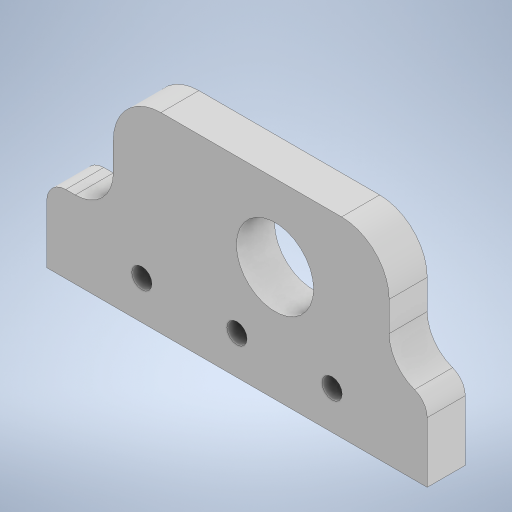
# Autodesk Inventor part: bottomhingeholder
Saved by Autodesk Inventor 2024 (Build 280153000, 153)
## iProperties
Created: 2023-09-15
Part Number: bottomhingeholder
Material: Generic
Document SubType Name: Modeling
Designer: komor
Density: 1 g/cm^3
Appearance: Default
Author: komor
Autodesk Inventor part; units mm, degrees
ref_plane "YZ Plane" through (0, 0, 0) normal (1, 0, 0) x (0, 1, 0)
ref_plane "XZ Plane" through (0, 0, 0) normal (0, 1, 0) x (-1, 0, 0)
ref_plane "XY Plane" through (0, 0, 0) normal (0, 0, 1) x (1, 0, 0)
sketch "Sketch1" plane through (0, 0, 0) normal (0, 0, 1) x (1, 0, 0)
  line L0 (30.5843, 30.8924) -> (30.5843, 10.8924)
  line L1 (30.5843, 10.8924) -> (-69.4157, 10.8924)
  line L2 (-69.4157, 10.8924) -> (-69.4157, 31.1924)
  line L3 (-69.4157, 21.0424) -> (30.5843, 20.8924) construction
  line L4 (-9.4157, 61.1924) -> (-39.4157, 61.1924)
  line L5 (-51.9157, 48.6924) -> (-51.9157, 41.1924)
  arc A0 (-39.4157, 61.1924) -> (-51.9157, 48.6924) centre (-39.4157, 48.6924) ccw
  line L6 (30.5843, 30.8924) -> (30.5843, 30.8924)
  line L7 (-61.9157, 31.1924) -> (-69.4157, 31.1924)
  arc A1 (-61.9157, 31.1924) -> (-51.9157, 41.1924) centre (-61.9157, 41.1924) ccw
  circle A2 centre (-19.4157, 20.9674) radius 2.65
  line L8 (-69.4157, 21.0424) -> (-19.4157, 20.9674) construction
  line L9 (-19.4157, 20.9674) -> (30.5843, 20.8924) construction
  circle A3 centre (-44.4157, 21.0049) radius 2.65
  circle A4 centre (5.5843, 20.9299) radius 2.65
  line L10 (-9.4157, 51.1924) -> (-9.4157, 30.8924) construction
  line L11 (-9.4157, 51.1924) -> (-9.4157, 30.8924) construction
  circle A5 centre (-9.4157, 41.0424) radius 10.15
  line L12 (-9.4157, 61.1924) -> (8.0843, 61.1924)
  line L13 (20.5843, 48.6924) -> (20.5843, 40.8924)
  arc A6 (20.5843, 48.6924) -> (8.0843, 61.1924) centre (8.0843, 48.6924) ccw
  arc A7 (20.5843, 40.8924) -> (30.5843, 30.8924) centre (30.5843, 40.8924) ccw
  point P0 (0, 0)
  point P1 (20.5843, 61.1924)
  point P2 (30.5843, 30.8924)
  dimension "d0" = 100
  dimension "d1" = 20
  dimension "d2" = 20.3
  dimension "d6" = 10
  dimension "d9" = 12.5
  dimension "d10" = 30
  dimension "d11" = 10
  dimension "d12" = 40
  dimension "d13" = 5.3
  dimension "d14" = 5.3
  dimension "d15" = 5.3
  dimension "d18" = 30
  dimension "d19" = 12.5
  dimension "d20" = 10
  constraints: 28 end point, 9 tangent, 8 centre point, 8 point on circle, 6 midpoint, 3 horizontal, 3 point on line, 2 collinear, 2 parallel, 1 perpendicular, 1 vertical
  measures "d0" distance of L0.end L1.end
  measures "d1" distance of L0.start L0.end
  measures "d2" distance of L10.end L10.start
  measures "d6" distance of L10.start L4.start
  measures "d9" radius of A0
  measures "d10" distance of L4.start L4.end
  measures "d11" radius of A1
  measures "d12" distance of L0.start L10.end
  measures "d13" diameter of A2
  measures "d14" diameter of A3
  measures "d15" diameter of A4
  measures "d18" distance of L4.start point (20.584, 61.192)
  measures "d19" radius of A6
  measures "d20" radius of A7
extrude "Extrusion1" add sketch "Sketch1" against normal blind 10
fillet "Fillet1" radius 5 2 edges at (-69.4157, 31.1924, -5) (30.5843, 30.8924, -5)
body "Solid1"
